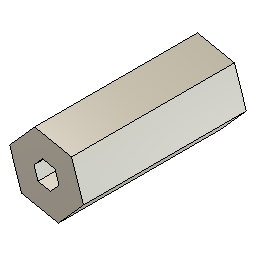
MondoHex+Long (Autodesk Fusion 360 design; units mm, degrees)
Autodesk Fusion 360 part; units mm, degrees
sketch "Sketch1" plane through (0, 0, 0) normal (0, 0, 1) x (1, 0, 0)
  line L0 (4.9621, 5.5958) -> (-2.3651, 7.0952)
  line L1 (-2.3651, 7.0952) -> (-7.3272, 1.4994)
  line L2 (-7.3272, 1.4994) -> (-4.9621, -5.5958)
  line L3 (-4.9621, -5.5958) -> (2.3651, -7.0952)
  line L4 (2.3651, -7.0952) -> (7.3272, -1.4994)
  line L5 (7.3272, -1.4994) -> (4.9621, 5.5958)
  line L6 (-6.9561, 20.8682) -> (-21.5505, 4.41)
  line L7 (-21.5505, 4.41) -> (-14.5944, -16.4583)
  line L8 (-14.5944, -16.4583) -> (6.9561, -20.8682)
  line L9 (6.9561, -20.8682) -> (21.5505, -4.41)
  line L10 (21.5505, -4.41) -> (14.5944, 16.4583)
  line L11 (14.5944, 16.4583) -> (-6.9561, 20.8682)
  dimension "d1" = 6.477
  dimension "d2" = 12.573
  measures "d1" distance of origin L5
extrude "Extrude1" add sketch "Sketch1" along normal blind 95.25
equation "d2 = 0.75 in - d1"
